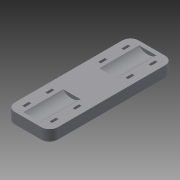
# Autodesk Inventor part: Y BEARING BLOCK
Saved by Autodesk Inventor 2013 (Build 170138000, 138)
## iProperties
Created: 2014-03-04
Part Number: Y BEARING BLOCK
Material: Generic
Document SubType Name: Modeling
Designer: employee
Density: 1 g/cm^3
Author: employee
Autodesk Inventor part; units mm, degrees
ref_plane "YZ Plane" through (0, 0, 0) normal (1, 0, 0) x (0, 1, 0)
ref_plane "XZ Plane" through (0, 0, 0) normal (0, 1, 0) x (-1, 0, 0)
ref_plane "XY Plane" through (0, 0, 0) normal (0, 0, 1) x (1, 0, 0)
sketch "Sketch1" plane through (0, 0, 0) normal (0, 0, 1) x (1, 0, 0)
  line L0 (-13, 37.5) -> (13, 37.5)
  line L1 (13, 37.5) -> (13, -37.5)
  line L2 (13, -37.5) -> (-13, -37.5)
  line L3 (-13, -37.5) -> (-13, 37.5)
  point P0 (0, 0)
  point P1 (-13, 0)
  point P2 (0, 37.5)
  dimension "d0" = 26
  dimension "d2" = 75
  constraints: 8 end point, 2 midpoint, 2 parallel, 1 horizontal, 1 horizontal alignment, 1 perpendicular, 1 vertical alignment
  measures "d0" distance of L1.end L2.end
  measures "d2" distance of L0.end L1.end
extrude "Extrusion1" add sketch "Sketch1" along normal blind 6.477
sketch "Sketch2" plane through (0, 0, 6.477) normal (0, 0, 1) x (1, 0, 0)
  line L0 (13, 37.5) -> (-13, 37.5) projected
  line L1 (-5.3033, 35) -> (5.3033, 35)
  line L2 (5.3033, 35) -> (5.3033, 11)
  line L3 (5.3033, 11) -> (-5.3033, 11)
  line L4 (-5.3033, 11) -> (-5.3033, 35)
  circle A0 centre (0, 35) radius 7.5
  line L5 (0, 35) -> (5.3033, 29.6967)
  point P0 (0, 0)
  point P1 (0, 37.5)
  dimension "d7" = 15
  dimension "d5" = 35
  dimension "d6" = 45
  dimension "d8" = 24
  constraints: 10 end point, 2 midpoint, 2 parallel, 1 coincident, 1 horizontal, 1 perpendicular, 1 point on line, 1 vertical alignment, 3 other
  measures "d5" distance from line of L1 point (0, 0)
  measures "d6" angle of L1 L5
  measures "d8" distance of L1.end L2.end
extrude "Extrusion2" cut sketch "Sketch2" against normal through all contours A0 L2 L3 L4 | L4 L1 L5 A0 | L5 L1 L2
sketch "Sketch3" plane through (0, 0, 6.477) normal (0, 0, 1) x (1, 0, 0)
  line L0 (-5.3033, 11) -> (-5.3033, 35) projected
  line L1 (-5.3033, 35) -> (5.3033, 35) projected
  line L2 (-7.5, 28) -> (7.5, 28) construction
  line L3 (7.5, 28) -> (7.5, 18) construction
  line L4 (7.5, 18) -> (-7.5, 18) construction
  line L5 (-7.5, 18) -> (-7.5, 28) construction
  line L6 (-7.5, 28) -> (-9, 28)
  line L7 (-9, 28) -> (-9, 32)
  line L8 (-9, 32) -> (-7.5, 32)
  line L9 (-7.5, 32) -> (-7.5, 28)
  line L10 (7.5, 28) -> (9, 28)
  line L11 (9, 28) -> (9, 32)
  line L12 (9, 32) -> (7.5, 32)
  line L13 (7.5, 32) -> (7.5, 28)
  line L14 (7.5, 18) -> (9, 18)
  line L15 (9, 18) -> (9, 14)
  line L16 (9, 14) -> (7.5, 14)
  line L17 (7.5, 14) -> (7.5, 18)
  line L18 (-7.5, 18) -> (-9, 18)
  line L19 (-9, 18) -> (-9, 14)
  line L20 (-9, 14) -> (-7.5, 14)
  line L21 (-7.5, 14) -> (-7.5, 18)
  point P0 (0, 0)
  point P1 (0, 28)
  point P2 (0, 35)
  point P3 (-7.5, 23)
  point P4 (-5.3033, 23)
  point P5 (-7.5, 30)
  dimension "d11" = 4
  dimension "d13" = 1.5
  dimension "d14" = 15
  dimension "d15" = 5
  constraints: 40 end point, 10 parallel, 6 equal length, 5 horizontal, 5 midpoint, 5 perpendicular, 1 horizontal alignment, 1 vertical alignment
  measures "d11" distance of L12.end L2.end
  measures "d13" distance of L2.end L10.end
  measures "d14" distance between parallel lines of L13 L9
  measures "d15" distance from line of L1 point (-7.5, 30)
extrude "Extrusion3" cut sketch "Sketch3" against normal through all
mirror "Mirror1" about plane through (0, 0, 0) normal (0, 1, 0) of "Extrusion3", "Extrusion2"
sketch "Sketch4" plane through (-5.3033, 35, 6.477) normal (0, -1, 0) x (1, 0, 0)
  line L0 (10.6066, -6.477) -> (0, -6.477) projected
  line L1 (10.6066, 0) -> (10.6066, -6.477) projected
  line L2 (0, 0) -> (10.6066, 0) projected
  line L3 (0, 0) -> (0, -6.477) projected
  arc A0 (0, 0) -> (10.6066, 0) centre (5.3033, 5.3033) ccw
  point P0 (5.3033, -6.477)
  dimension "d18" = 15
  constraints: 2 end point, 2 point on circle, 1 centre point
  measures "d18" diameter of A0
extrude "Extrusion4" add sketch "Sketch4" along normal up to surface (70 mm away) contours L0 L3 A0 L1
fillet "Fillet1" radius 5 4 edges at (13, -37.5, 3.2385) (13, 37.5, 3.2385) (-13, 37.5, 3.2385) (-13, -37.5, 3.2385)
body "Solid1"
